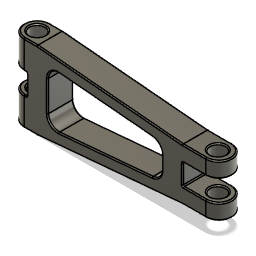
upper link v1 (Autodesk Fusion 360 archive; units mm, degrees)
design "new upper link"
Autodesk Fusion 360 part; units mm, degrees
sketch "Sketch1" plane through (0, 0, 0) normal (0, 0, 1) x (1, 0, 0)
  line L0 (-25, 0) -> (-25, 10)
  line L1 (-25, 10) -> (-40, 10)
  line L2 (-40, 10) -> (-40, 37.5)
  line L3 (-40, 37.5) -> (-15, 37.5)
  line L4 (-15, 37.5) -> (125, 25)
  line L5 (125, 25) -> (160, 25)
  line L6 (160, 25) -> (160, 10)
  line L7 (160, 10) -> (125, 10)
  line L8 (125, 10) -> (125, 0)
  line L9 (-5, 25.648) -> (105, 15.8266)
  line L10 (-5, 25.648) -> (-5, 0)
  line L11 (105, 15.8266) -> (105, 0)
  line L12 (-65, 0) -> (170, 0) construction
  line L13 (-40, -10) -> (-40, -37.5)
  line L14 (-15, -37.5) -> (125, -25)
  line L15 (-25, -10) -> (-40, -10)
  line L16 (125, -25) -> (160, -25)
  line L17 (-5, -25.648) -> (105, -15.8266)
  line L18 (-5, -25.648) -> (-5, 0)
  line L19 (-40, -37.5) -> (-15, -37.5)
  line L20 (-65, 0) -> (170, 0) construction
  line L21 (-25, 0) -> (-25, -10)
  line L22 (105, -15.8266) -> (105, 0)
  line L23 (160, -25) -> (160, -10)
  line L24 (160, -10) -> (125, -10)
  line L25 (125, -10) -> (125, 0)
  dimension "d1" = 10
  dimension "d2" = 27.5
  dimension "d3" = 25
  dimension "d4" = 200
  dimension "d5" = 10
  dimension "d6" = 15
  dimension "d7" = 35
  dimension "d8" = 35
  dimension "d9" = 20
  dimension "d10" = 20
  constraint vertical L0
  constraint perpendicular L0 L1
  constraint perpendicular L1 L2
  constraint perpendicular L2 L3
  constraint perpendicular L2 L5
  constraint perpendicular L5 L6
  constraint perpendicular L2 L7
  constraint perpendicular L7 L8
  constraint parallel L4 L9
  constraint perpendicular L3 L10
  constraint vertical L11
  constraint horizontal L12
  constraint symmetric L0.start L12 L21.start
  constraint symmetric L0.end L12 L15.start
  constraint symmetric L1.end L12 L13.start
  constraint symmetric L2.end L12 L13.end
  constraint symmetric L3.end L12 L14.start
  constraint symmetric L4.end L12 L14.end
  constraint symmetric L5.end L12 L16.end
  constraint symmetric L6.end L12 L23.end
  constraint symmetric L7.end L12 L24.end
  constraint symmetric L8.end L12 L25.end
  constraint symmetric L9.start L12 L17.start
  constraint symmetric L9.end L12 L17.end
  constraint symmetric L10.end L12 L18.end
  constraint symmetric L11.end L12 L22.end
  constraint symmetric L20.start L12 L12.start
  constraint symmetric L20.end L12 L12.end
  measures "d1" distance of L0.start L0.end
  measures "d2" distance of L1.end L2.end
  measures "d3" distance of L2.end L3.end
  measures "d4" distance of L2 L6
  measures "d5" distance of L7.end L8.end
  measures "d6" distance of L5.end L6.end
  measures "d7" distance of L4.end L5.end
  measures "d8" distance of L6.end L7.end
  measures "d9" horizontal distance of L0.end L9.start
  measures "d10" horizontal distance of L7.end L9.end
extrude "Extrude1" add sketch "Sketch1" along normal blind 12.5 and the other way blind 12.5
fillet "Fillet1" radius 12.5 8 edges at (160, 17.5, 12.5) (160, 17.5, -12.5) (160, -17.5, -12.5) (160, -17.5, 12.5) (-40, -23.75, 12.5) (-40, 23.75, 12.5) (-40, 23.75, -12.5) (-40, -23.75, -12.5)
fillet "Fillet2" radius 10 4 edges at (-5, -25.648, 0) (-5, 25.648, 0) (105, 15.8266, 0) (105, -15.8266, 0)
sketch "Sketch2" plane through (0, 37.5, 0) normal (0, 1, 0) x (-1, 0, 0)
  arc A0 (27.5, -12.5) -> (27.5, 12.5) centre (27.5, 0) ccw
  line L0 (27.5, 12.5) -> (15, 12.5)
  line L1 (15, 12.5) -> (15, -12.5)
  line L2 (15, -12.5) -> (27.5, -12.5)
  circle A1 centre (27.5, 0) radius 7.5
  circle A2 centre (-146.5, 0) radius 7.5
  dimension "d19" = 15
  dimension "d20" = 15
  constraint coincident A0.centre A1.centre
  measures "d19" diameter of A1
  measures "d20" diameter of A2
extrude "Extrude2" cut sketch "Sketch2" along normal blind 0 and the other way blind 80 contours A1 | A2
fillet "Fillet3" radius 1 60 edges at (50.8893, 20.6579, 12.5) (-1.7493, 22.0942, 12.5) (-5, 0, 12.5) (-1.7493, -22.0942, 12.5) (50.8893, -20.6579, 12.5) (102.3788, -13.429, 12.5) (105, 0, 12.5) (102.3788, 13.429, 12.5) (55, 31.25, -12.5) (-21.25, -37.5, -12.5) (-40, -37.5, 0) (-21.25, -37.5, 12.5) (-25, 10, -9.7855) (-25, -10, -9.7855) (-25, -10, 9.7855) (-15, 37.5, 0) (125, 10, 0) (-26.25, -10, 12.5) (-40, -10, 0) (-26.25, -10, -12.5) (125, -25, 0) (-26.25, 10, -12.5) (-40, 10, 0) (-26.25, 10, 12.5) (-21.25, 37.5, 12.5) (-40, 37.5, 0) (-21.25, 37.5, -12.5) (125, 0, 12.5) (125, 25, 0) (136.25, 10, 12.5) (160, 10, 0) (136.25, 10, -12.5) (-25, 0, -7.0711) (55, -31.25, -12.5) (-1.7493, 22.0942, -12.5) (-5, 0, -12.5) (-1.7493, -22.0942, -12.5) (50.8893, -20.6579, -12.5) (102.3788, -13.429, -12.5) (105, 0, -12.5) (102.3788, 13.429, -12.5) (50.8893, 20.6579, -12.5) (55, -31.25, 12.5) (-25, 10, 9.7855) (-15, -37.5, 0) (55, 31.25, 12.5) (136.25, 25, -12.5) (160, 25, 0) (136.25, 25, 12.5) (125, -10, 0) (-25, 0, 7.0711) (-25, 0, 12.5) (136.25, -25, 12.5) (160, -25, 0) (136.25, -25, -12.5) (136.25, -10, -12.5) (160, -10, 0) (136.25, -10, 12.5) (125, 0, -12.5) (-25, 0, -12.5) 38 faces at (5.4293, 24.7061, -4.1667) (35.8893, 21.9972, 4.1667) (98.2972, 16.1204, 4.1667) (105, 2.2266, 4.1667) (96.8673, -16.5038, 4.1667) (35.8893, -21.9972, 4.1667) (4.9684, -24.7153, 4.1667) (-5, -4.9051, 4.1667) (129.6667, -25, 0) (139.0373, 15, -0.7468) (-11.6667, -3.3333, -12.5) (-39.9434, -19.1667, 1.1905) (-39.9434, -19.1667, -1.1905) (-40, -19.1667, 0.0008) (-11.6667, -3.3333, 12.5) (-39.9434, 19.1667, 1.1905) (-33.2292, 28.3333, -11.1107) (-40, 19.1667, 0.0008) (155.2279, -20, 9.8262) (160, -15, 0.0008) (159.9858, -20, -0.5972) (159.9858, 20, 0.5972) (160, 15, 0.0008) (155.2279, 20, -9.8262) (31.6667, 33.3333, -4.1667) (31.6667, -33.3333, -4.1667) (139.0373, -20, -0.7468) (-22.0842, 37.5, 10.4984) (-26.1883, 10, -10.787) (-24.1546, -3.3333, 6.7126) (129.6667, 10, 0) (125, 3.3333, -4.1667) (-25, 3.3333, 8.8807) (129.6667, -10, 0) (-25, 3.3333, -8.8807) (129.6667, 25, 0) (-22.0842, -37.5, -10.4984) (-26.1883, -10, -10.787)
